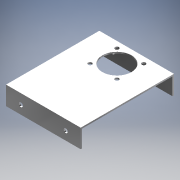
# Autodesk Inventor part: Spacer Extrusion
Saved by Autodesk Inventor 2019 (Build 230136000, 136)
## iProperties
Created: 2019-10-20
Part Number: Spacer Extrusion
Material: Aluminum 6061
Document SubType Name: Modeling
Designer: admin
Density: 2.7 g/cm^3
Appearance: Aluminum - Flat
Author: admin
Autodesk Inventor part; units mm, degrees
ref_plane "YZ Plane" through (0, 0, 0) normal (1, 0, 0) x (0, 1, 0)
ref_plane "XZ Plane" through (0, 0, 0) normal (0, 1, 0) x (-1, 0, 0)
ref_plane "XY Plane" through (0, 0, 0) normal (0, 0, 1) x (1, 0, 0)
sketch "Sketch1" plane through (0, 0, 0) normal (1, 0, 0) x (0, 1, 0)
  line L0 (0, 0) -> (25, 0)
  line L1 (25, 0) -> (25, -125)
  line L2 (25, -125) -> (0, -125)
  line L3 (0, -125) -> (0, -123)
  line L4 (0, -123) -> (23, -123)
  line L5 (23, -123) -> (23, -2)
  line L6 (23, -2) -> (0, -2)
  line L7 (0, -2) -> (0, 0)
  dimension "d0" = 2
  dimension "d1" = 2
  dimension "d2" = 125
  dimension "d3" = 25
  dimension "d4" = 2
  constraints: 16 end point, 7 perpendicular, 1 horizontal, 1 point on line
  measures "d0" distance of L6.end L0.start
  measures "d1" distance of L2.end L3.end
  measures "d2" distance of L0.end L1.end
  measures "d3" distance of L0.start L0.end
  measures "d4" distance between parallel lines of L1 L5
extrude "Extrusion1" add sketch "Sketch1" along normal blind 100
sketch "Sketch2" plane through (0, 0, -123) normal (0, 0, 1) x (1, 0, 0)
  circle A0 centre (80, 11.5) radius 2.75
  line L0 (0, 23) -> (100, 23) projected
  line L1 (100, 23) -> (100, 0) projected
  circle A1 centre (20, 11.5) radius 2.75
  line L2 (0, 0) -> (100, 0) projected
  line L3 (0, 0) -> (0, 23) projected
  dimension "d7" = 5.5
  dimension "d8" = 11.5
  dimension "d9" = 20
  dimension "d10" = 5.5
  dimension "d11" = 11.5
  dimension "d12" = 20
  constraints: 2 centre point
  measures "d7" diameter of A0
  measures "d8" distance from line of L0 A0.centre
  measures "d9" distance from line of A0.centre L1
  measures "d10" diameter of A1
  measures "d11" distance from line of L2 A1.centre
  measures "d12" distance from line of L3 A1.centre
extrude "Extrusion2" cut sketch "Sketch2" along normal blind 139.25 and the other way blind 73.375 contours A0 | A1
sketch "Sketch3" plane through (0, 25, 0) normal (0, 1, 0) x (1, 0, 0)
  circle A0 centre (67.9615, 116.548) radius 2.6
  line L0 (0, 125) -> (100, 125) projected
  circle A1 centre (32.0385, 116.548) radius 2.6
  circle A2 centre (67.9615, 80.625) radius 2.6
  circle A3 centre (32.0385, 80.625) radius 2.6
  line L1 (100, 125) -> (100, 0) projected
  circle A4 centre (50, 98.5865) radius 19.5
  line L2 (67.9615, 116.548) -> (32.0385, 80.625)
  line L3 (32.0385, 116.548) -> (67.9615, 80.625)
  circle A5 centre (50, 33.813) radius 32.5
  line L4 (0, 0) -> (100, 0) projected
  dimension "d17" = 5.2
  dimension "d18" = 8.452
  dimension "d19" = 5.2
  dimension "d20" = 5.2
  dimension "d21" = 5.2
  dimension "d22" = 35.923
  dimension "d23" = 35.923
  dimension "d24" = 35.923
  dimension "d25" = 35.923
  dimension "d26" = 32.0385
  dimension "d27" = 32.0385
  dimension "d28" = 8.452
  dimension "d31" = 39
  dimension "d32" = 65
  dimension "d33" = 33.813
  dimension "d34" = 50
  constraints: 6 centre point, 4 end point, 2 midpoint
  measures "d17" diameter of A0
  measures "d18" distance from line of L2.start L0
  measures "d19" diameter of A1
  measures "d20" diameter of A2
  measures "d21" diameter of A3
  measures "d22" distance of L2.start L3.end
  measures "d23" distance of L3.end L2.end
  measures "d24" distance of L2.start L3.start
  measures "d25" distance of L2.end L3.start
  measures "d26" distance from line of L1 L2.start
  measures "d27" distance from line of L1 L3.end
  measures "d28" distance from line of L0 L3.start
  measures "d31" diameter of A4
  measures "d32" diameter of A5
  measures "d33" distance from line of L4 A5.centre
  measures "d34" distance from line of L1 A5.centre
extrude "Extrusion3" cut sketch "Sketch3" against normal blind 10
body "Solid1"
